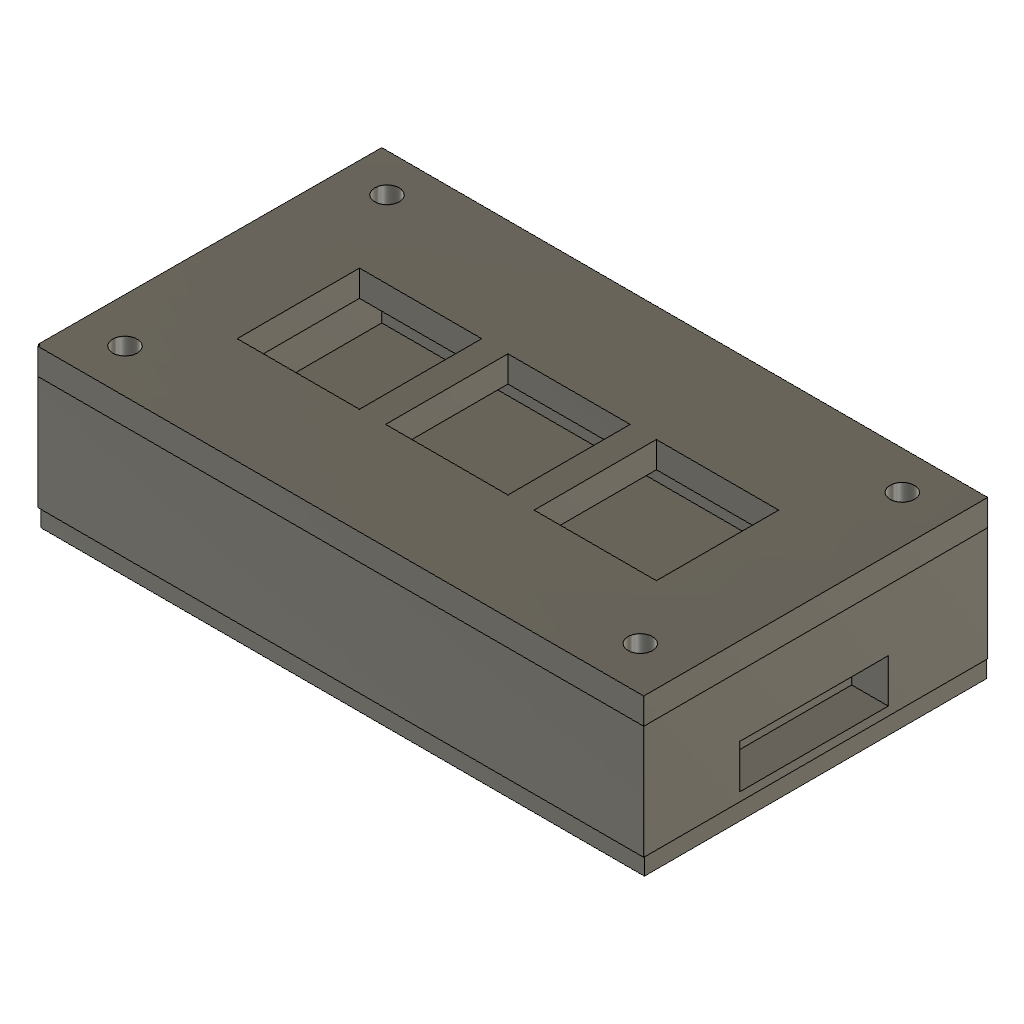
F3D UPDATED (Autodesk Fusion 360 design; units mm, degrees)
part number: 2026-07-22-23-07-19-402
Autodesk Fusion 360 part; units mm, degrees
form "Form1" [no effect]
sketch "sketch 359" plane through (0, 0, 0) normal (0, 0, 1) x (1, 0, 0)
  line L0 (0, 0) -> (49.4, 0)
  line L1 (49.4, 0) -> (49.4, 19.4)
  line L2 (49.4, 19.4) -> (0, 19.4)
  line L3 (0, 19.4) -> (0, 0)
  line L4 (-10, 29.4) -> (59.4, 29.4)
  line L5 (59.4, 29.4) -> (59.4, -10)
  line L6 (59.4, -10) -> (-10, -10)
  line L7 (-10, -10) -> (-10, 29.4)
  circle A0 centre (-5, 25) radius 1.45
  circle A1 centre (54, 25) radius 1.45
  circle A2 centre (54, -5) radius 1.45
  circle A3 centre (-5, -5) radius 1.45
  constraint horizontal L0
  constraint vertical L1
  constraint horizontal L2
  constraint vertical L3
  constraint coincident L0.start L3.end
  constraint horizontal L4
  constraint vertical L5
  constraint horizontal L6
  constraint vertical L7
extrude "Extrude1" add sketch "sketch 359" along normal blind 3 makes body 1
extrude "Extrude2" add 1 faces at (16.3333, 23.5528, 3) along direction (0, 0, 1) blind 10 on bodies 1 bodies 1
sketch "Sketch1" plane through (0, 0, 0) normal (0, 0, 1) x (1, 0, 0)
  line L0 (59.352, 29) -> (-10, 29)
  line L1 (-10, 29) -> (-10, -9.736)
  line L2 (-10, -9.736) -> (59.352, -9.736)
  line L3 (59.352, -9.736) -> (59.352, 29)
  constraint horizontal L0
  constraint vertical L1
  constraint horizontal L2
  constraint vertical L3
extrude "Extrude3" add sketch "Sketch1" along normal blind 3 bodies 1
extrude "Extrude4" cut sketch "sketch 359" along normal through all contours A0 | A1 | A2 | A3 bodies 1
sketch "Sketch2" plane through (0, 0, 3) normal (0, 0, 1) x (-1, 0, 0)
  line L0 (0, 0) -> (-49.4, 0)
  line L1 (-49.4, 0) -> (-49.4, -19.4)
  line L2 (-49.4, -19.4) -> (0, -19.4)
  line L3 (0, -19.4) -> (0, 0)
sketch "Sketch3" plane through (0, 0, 0) normal (0, 0, 1) x (1, 0, 0)
sketch "sketch 3672" plane through (0, 0, 0) normal (0, 0, 1) x (1, 0, 0)
  line L0 (14.5, 16) -> (14.5, 3)
  line L1 (3.0489, 16.475) -> (14, 16.5)
  line L2 (3.025, 2.3766) -> (14, 2.5)
  line L3 (2.5489, 15.975) -> (2.525, 2.8766)
  line L4 (35.3489, 16.4816) -> (46.1543, 16.5621)
  arc A0 (14.5, 16) -> (14, 16.5) centre (14, 16) ccw
  line L5 (30.5, 16) -> (30.5, 3)
  arc A1 (18.5, 3) -> (19, 2.5) centre (19, 3) ccw
  line L6 (18.5, 16) -> (18.5, 3)
  line L7 (35.5886, 2.1369) -> (46.2741, 2.1163)
  line L8 (34.8489, 15.9816) -> (35.0886, 2.6369)
  arc A2 (14, 2.5) -> (14.5, 3) centre (14, 3) ccw
  line L9 (46.6543, 16.0621) -> (46.7741, 2.6163)
  arc A3 (2.525, 2.8766) -> (3.025, 2.3766) centre (3.025, 2.8766) ccw
  arc A4 (3.0489, 16.475) -> (2.5489, 15.975) centre (3.0489, 15.975) ccw
  line L10 (19, 16.5) -> (30, 16.5)
  arc A5 (30.5, 16) -> (30, 16.5) centre (30, 16) ccw
  line L11 (19, 2.5) -> (30, 2.5)
  arc A6 (19, 16.5) -> (18.5, 16) centre (19, 16) ccw
  arc A7 (30, 2.5) -> (30.5, 3) centre (30, 3) ccw
  arc A8 (35.3489, 16.4816) -> (34.8489, 15.9816) centre (35.3489, 15.9816) ccw
  arc A9 (35.0886, 2.6369) -> (35.5886, 2.1369) centre (35.5886, 2.6369) ccw
  arc A10 (46.6543, 16.0621) -> (46.1543, 16.5621) centre (46.1543, 16.0621) ccw
  arc A11 (46.2741, 2.1163) -> (46.7741, 2.6163) centre (46.2741, 2.6163) ccw
  line L12 (-10.0721, -9.8522) -> (-9.8977, 29.2855)
  line L13 (59, -10) -> (59, 29)
  line L14 (-9.8977, 29.2855) -> (59, 29)
  line L15 (-10.0721, -9.8522) -> (59, -10)
extrude "Extrude5" add sketch "sketch 3672" against normal blind 3 separate body makes body 2
sketch "Sketch4" plane through (59.4, 0, 0) normal (1, 0, 0) x (0, 1, 0)
  line L0 (-10, 0) -> (29.4, 0)
  line L1 (29.4, 0) -> (29.4, 13)
  line L2 (29.4, 13) -> (-10, 13)
  line L3 (-10, 13) -> (-10, 0)
  line L4 (1, 9) -> (18, 9)
  line L5 (18, 9) -> (18, 4)
  line L6 (18, 4) -> (1, 4)
  line L7 (1, 4) -> (1, 9)
  dimension "d10" = 5
  dimension "d11" = 17
  constraint horizontal L4
  constraint vertical L5
  constraint horizontal L6
  constraint vertical L7
  measures "d10" distance of L4.end L5.end
  measures "d11" distance of L4.start L4.end
extrude "Extrude6" cut sketch "Sketch4" against normal blind 10 contours L4 L5 L6 L7 bodies 1
sketch "Sketch5" plane through (0, 0, 13) normal (0, 0, 1) x (-1, 0, 0)
  line L0 (0, 0) -> (0, -19.4)
  line L1 (0, -19.4) -> (-49.4, -19.4)
  line L2 (-49.4, -19.4) -> (-49.4, 0)
  line L3 (-49.4, 0) -> (0, 0)
  circle A0 centre (-54, 5) radius 1.45
  circle A1 centre (5, 5) radius 1.45
  circle A2 centre (5, -25) radius 1.45
  circle A3 centre (-54, -25) radius 1.45
  line L4 (10, 10) -> (-59.4, 10)
  line L5 (-59.4, 10) -> (-59.4, -29.4)
  line L6 (-59.4, -29.4) -> (10, -29.4)
  line L7 (10, -29.4) -> (10, 10)
sketch "Sketch6" plane through (0, 0, -3) normal (0, 0, -1) x (1, 0, 0)
  arc A0 (18.5, -16) -> (19, -16.5) centre (19, -16) ccw
  line L0 (18.5, -16) -> (18.5, -3)
  arc A1 (19, -2.5) -> (18.5, -3) centre (19, -3) ccw
  line L1 (19, -2.5) -> (30, -2.5)
  arc A2 (30.5, -3) -> (30, -2.5) centre (30, -3) ccw
  line L2 (30.5, -3) -> (30.5, -16)
  arc A3 (30, -16.5) -> (30.5, -16) centre (30, -16) ccw
  line L3 (30, -16.5) -> (19, -16.5)
  arc A4 (34.8489, -15.9816) -> (35.3489, -16.4816) centre (35.3489, -15.9816) ccw
  line L4 (34.8489, -15.9816) -> (35.0886, -2.6369)
  arc A5 (35.5886, -2.1369) -> (35.0886, -2.6369) centre (35.5886, -2.6369) ccw
  line L5 (35.5886, -2.1369) -> (46.2741, -2.1163)
  arc A6 (46.7741, -2.6163) -> (46.2741, -2.1163) centre (46.2741, -2.6163) ccw
  line L6 (46.7741, -2.6163) -> (46.6543, -16.0621)
  arc A7 (46.1543, -16.5621) -> (46.6543, -16.0621) centre (46.1543, -16.0621) ccw
  line L7 (46.1543, -16.5621) -> (35.3489, -16.4816)
  arc A8 (14, -16.5) -> (14.5, -16) centre (14, -16) ccw
  line L8 (14, -16.5) -> (3.0489, -16.475)
  arc A9 (2.5489, -15.975) -> (3.0489, -16.475) centre (3.0489, -15.975) ccw
  line L9 (2.5489, -15.975) -> (2.525, -2.8766)
  arc A10 (3.025, -2.3766) -> (2.525, -2.8766) centre (3.025, -2.8766) ccw
  line L10 (3.025, -2.3766) -> (14, -2.5)
  arc A11 (14.5, -3) -> (14, -2.5) centre (14, -3) ccw
  line L11 (14.5, -3) -> (14.5, -16)
  line L12 (-10.0721, 9.8522) -> (-9.8977, -29.2855)
  line L13 (-9.8977, -29.2855) -> (59, -29)
  line L14 (59, -29) -> (59, 10)
  line L15 (59, 10) -> (-10.0721, 9.8522)
move_face "MoveFace1" by (-60, 0, 0) 1 faces at (16.3333, 23.5528, 13) on bodies 1
move_face "MoveFace2" to x (0.939693, -0.34202, 0) y (0.34202, 0.939693, 0) z (0, 0, 1) at (-4.6871, -1.2103, -13) 2 faces at (32.9333, 6.4667, 3) (16.3333, 23.5528, 13) on bodies 1
move_body "Move1" bodies 1 to x (1, 0, 0) y (0, 1, 0) z (0, 0, 1) at (-70.6858, -0.1603, 0)
extrude "Extrude7" cut 1 faces at (-36.7879, 5.0494, 0) along direction (0, 0, 1) blind 3 on bodies 1 bodies 1
extrude "Extrude8" add 1 faces at (-54.3524, 23.3925, 13) along direction (0, 0, 1) blind 3 on bodies 1 bodies 1
move_face "MoveFace3" by (-60.7884, -19.4774, 0) 1 faces at (26.3674, 24.9285, 0) on bodies 2
move_face "MoveFace4" by (80, 0, 0) 1 faces at (-54.3524, 23.3925, 16) on bodies 1
move_face "MoveFace5" by (0, 0, 25) 1 faces at (12.9519, -9.9014, -1) on bodies 2
sketch "Sketch7" plane through (0, -10.1603, 0) normal (0, -1, 0) x (1, 0, 0)
  line L0 (-80.6858, 3) -> (-11.2858, 3)
  line L1 (-11.2858, 3) -> (-11.2858, 16)
  line L2 (-11.2858, 16) -> (-80.6858, 16)
  line L3 (-80.6858, 16) -> (-80.6858, 3)
move_face "MoveFace6" by (70, 0, 0) 1 faces at (-54.3524, 23.3925, 16) on bodies 1
move_body "Move2" bodies 2 to x (1, 0, 0) y (0, 1, 0) z (0, 0, 1) at (-70.8, 0, 0)
move_face "MoveFace7" by (0, 0, 20) 1 faces at (-57.8481, -9.9014, -2) on bodies 2
move_body "Move3" bodies 2 to x (1, 0, 0) y (0, 1, 0) z (0, 0, 1) at (0.5, -0.0011, 19)
sketch "Sketch8" plane through (0, 0, 3) normal (0, 0, -1) x (1, 0, 0)
  line L0 (-21.2858, -19.2397) -> (-70.6858, -19.2397)
  line L1 (-70.6858, -19.2397) -> (-70.6858, 0.1603)
  line L2 (-70.6858, 0.1603) -> (-21.2858, 0.1603)
  line L3 (-21.2858, 0.1603) -> (-21.2858, -19.2397)
  circle A0 centre (-16.6858, -24.8397) radius 1.45
  circle A1 centre (-16.6858, 5.1603) radius 1.45
  circle A2 centre (-75.6858, -24.8397) radius 1.45
  circle A3 centre (-75.6858, 5.1603) radius 1.45
  line L4 (-80.6858, 10.1603) -> (-80.6858, -29.2397)
  line L5 (-80.6858, -29.2397) -> (-11.2858, -29.2397)
  line L6 (-11.2858, -29.2397) -> (-11.2858, 10.1603)
  line L7 (-11.2858, 10.1603) -> (-80.6858, 10.1603)
sketch "Sketch9" plane through (0, 0, 3) normal (0, 0, -1) x (1, 0, 0)
sketch "Sketch10" plane through (0, 0, 3) normal (0, 0, -1) x (1, 0, 0)
extrude "Extrude9" add sketch "Sketch8" against normal blind 0.01 contours L0 L1 L2 L3 bodies 1
move_body "Move4" bodies 2 to x (1, 0, 0) y (0, 1, 0) z (0, 0, 1) at (-0.3136, -0.3071, -3)
move_body "Move5" bodies 2 to x (1, 0, 0) y (0, 1, 0) z (0, 0, 1) at (-0.1744, 0.2623, 0)
hole "Hole1" at (-16.6858, 24.8397, 3) direction (0, 0, 1) diameter 2.8 depth 13 tip angle 118 bodies 2
hole "Hole2" at (-16.6858, -5.1603, 3) direction (0, 0, 1) diameter 2.8 depth 13 tip angle 118 bodies 2
hole "Hole3" at (-75.6858, -5.1603, 3) direction (0, 0, 1) diameter 2.8 depth 13 tip angle 118 bodies 2
hole "Hole4" at (-75.6858, 24.8397, 3) direction (0, 0, 1) diameter 2.8 depth 13 tip angle 118 bodies 2
sketch "Sketch11" plane through (0, 0, 16) normal (0, 0, 1) x (-1, 0, 0)
  circle A0 centre (75.6858, -24.8397) radius 1.4
  circle A1 centre (75.6858, 5.1603) radius 1.4
  circle A2 centre (16.6858, 5.1603) radius 1.4
  circle A3 centre (16.6858, -24.8397) radius 1.4
  arc A4 (51.788, -16.4542) -> (52.288, -15.9542) centre (51.788, -15.9542) ccw
  line L0 (51.788, -16.4542) -> (40.788, -16.4542)
  arc A5 (40.288, -15.9542) -> (40.788, -16.4542) centre (40.788, -15.9542) ccw
  line L1 (40.288, -15.9542) -> (40.288, -2.9542)
  arc A6 (40.788, -2.4542) -> (40.288, -2.9542) centre (40.788, -2.9542) ccw
  line L2 (40.788, -2.4542) -> (51.788, -2.4542)
  arc A7 (52.288, -2.9542) -> (51.788, -2.4542) centre (51.788, -2.9542) ccw
  line L3 (52.288, -2.9542) -> (52.288, -15.9542)
  arc A8 (35.4391, -16.4358) -> (35.9391, -15.9358) centre (35.4391, -15.9358) ccw
  line L4 (35.4391, -16.4358) -> (24.6337, -16.5163)
  arc A9 (24.1337, -16.0163) -> (24.6337, -16.5163) centre (24.6337, -16.0163) ccw
  line L5 (24.1337, -16.0163) -> (24.0139, -2.5705)
  arc A10 (24.5139, -2.0705) -> (24.0139, -2.5705) centre (24.5139, -2.5705) ccw
  line L6 (24.5139, -2.0705) -> (35.1994, -2.0911)
  arc A11 (35.6994, -2.5911) -> (35.1994, -2.0911) centre (35.1994, -2.5911) ccw
  line L7 (35.6994, -2.5911) -> (35.9391, -15.9358)
  arc A12 (56.288, -15.9542) -> (56.788, -16.4542) centre (56.788, -15.9542) ccw
  line L8 (56.288, -15.9542) -> (56.288, -2.9542)
  arc A13 (56.788, -2.4542) -> (56.288, -2.9542) centre (56.788, -2.9542) ccw
  line L9 (56.788, -2.4542) -> (67.763, -2.3308)
  arc A14 (68.263, -2.8308) -> (67.763, -2.3308) centre (67.763, -2.8308) ccw
  line L10 (68.263, -2.8308) -> (68.2391, -15.9292)
  arc A15 (67.7391, -16.4292) -> (68.2391, -15.9292) centre (67.7391, -15.9292) ccw
  line L11 (67.7391, -16.4292) -> (56.788, -16.4542)
  line L12 (80.6858, -29.2397) -> (80.8602, 9.898)
  line L13 (80.8602, 9.898) -> (11.788, 10.0458)
  line L14 (11.788, 10.0458) -> (11.788, -28.9542)
  line L15 (11.788, -28.9542) -> (80.6858, -29.2397)
  dimension "d36" = 12
  dimension "d45" = 14
  dimension "d49" = 14.3447
  dimension "d52" = 11.6855
  dimension "d53" = 14.0984
  dimension "d54" = 11.975
  dimension "d56" = 14.4463
  measures "d36" distance of L1 L3
  measures "d45" distance of L0 L2
  measures "d49" vertical distance of A8.start L6.end
  measures "d52" horizontal distance of L5.end A11.start
  measures "d53" vertical distance of L9.end A15.start
  measures "d54" horizontal distance of L8.end A14.start
  measures "d56" distance of L4.end A10.start
sketch "Sketch12" plane through (0, 0, 16) normal (0, 0, 1) x (-1, 0, 0)
  line L0 (70, -16) -> (56, -16)
  line L1 (56, -16) -> (56, -2)
  line L2 (56, -2) -> (70, -2)
  line L3 (70, -2) -> (70, -16)
  line L4 (22, -16) -> (36, -16)
  line L5 (36, -16) -> (36, -2)
  line L6 (36, -2) -> (22, -2)
  line L7 (22, -2) -> (22, -16)
  line L8 (53, -16) -> (39, -16)
  line L9 (39, -16) -> (39, -2)
  line L10 (39, -2) -> (53, -2)
  line L11 (53, -2) -> (53, -16)
  dimension "d57" = 14
  dimension "d58" = 14
  dimension "d59" = 14
  dimension "d60" = 14
  dimension "d61" = 14
  constraint horizontal L0
  constraint vertical L1
  constraint horizontal L2
  constraint vertical L3
  constraint horizontal L4
  constraint vertical L5
  constraint horizontal L6
  constraint vertical L7
  constraint horizontal L8
  constraint vertical L9
  constraint horizontal L10
  constraint vertical L11
  measures "d57" distance of L0.start L0.end
  measures "d58" distance of L4.start L4.end
  measures "d59" distance of L4.start L6.end
  measures "d60" distance of L8.start L8.end
  measures "d61" distance of L8.start L10.end
sketch "Sketch13" plane through (0, 0, 16) normal (0, 0, 1) x (-1, 0, 0)
  line L0 (73, -22) -> (15.4788, -22)
  line L1 (15.4788, -22) -> (15.4788, 2.4214)
  line L2 (15.4788, 2.4214) -> (73, 2.4214)
  line L3 (73, 2.4214) -> (73, -22)
  constraint horizontal L0
  constraint vertical L1
  constraint horizontal L2
  constraint vertical L3
extrude "Extrude10" add sketch "Sketch13" against normal blind 13 bodies 1 2
shell "Shell1" thickness 1.5 removed faces 1 at (-36.7879, 14.63, 3) on bodies 1
extrude "Extrude11" cut sketch "Sketch12" against normal blind 6 bodies 1
extrude "Extrude12" add 1 faces at (-48.4572, 22.5773, 16) along direction (0, 0, 1) blind 3 on bodies 1 bodies 1
sketch "Sketch14" plane through (0, 0, 0) normal (0, 0, 1) x (1, 0, 0)
  line L0 (-80.5, -10, 3) -> (-11.3436, -10, 3)
  line L1 (-11.3436, -10, 3) -> (-11.3436, 29.1649, 3)
  line L2 (-11.3436, 29.1649, 3) -> (-80.5, 29.1649, 3)
  line L3 (-80.5, 29.1649, 3) -> (-80.5, -10, 3)
  line L4 (-80.6858, -10.1603, 3) -> (-11.2858, -10.1603, 3)
  line L5 (-11.2858, -10.1603, 3) -> (-11.2858, 29.2397, 3)
  line L6 (-11.2858, 29.2397, 3) -> (-80.6858, 29.2397, 3)
  line L7 (-80.6858, 29.2397, 3) -> (-80.6858, -10.1603, 3)
  line L8 (-80.6858, -10.1603, 3) -> (-11.2858, -10.1603, 3)
  line L9 (-11.2858, -10.1603, 3) -> (-11.2858, 29.2397, 3)
  line L10 (-11.2858, 29.2397, 3) -> (-80.6858, 29.2397, 3)
  line L11 (-80.6858, 29.2397, 3) -> (-80.6858, -10.1603, 3)
  line L12 (-80.6858, -10.1603, 3) -> (-11.2858, -10.1603, 3)
  line L13 (-11.2858, -10.1603, 3) -> (-11.2858, 29.2397, 3)
  line L14 (-11.2858, 29.2397, 3) -> (-80.6858, 29.2397, 3)
  line L15 (-80.6858, 29.2397, 3) -> (-80.6858, -10.1603, 3)
  line L16 (-80.5, -10) -> (-11.3694, -10)
  line L17 (-11.3694, -10) -> (-11.3694, 29.2038)
  line L18 (-11.3694, 29.2038) -> (-80.5, 29.2038)
  line L19 (-80.5, 29.2038) -> (-80.5, -10)
  point P0 (-80.6858, -10.1603)
  point P1 (-11.2858, 29.2397)
  point P2 (-80.6858, -10.1603)
  point P3 (-11.2858, 29.2397)
  point P4 (-80.6858, -10.1603)
  point P5 (-11.2858, 29.2397)
  constraint coincident P5 P3
  constraint coincident P4 P2
  constraint horizontal L16
  constraint vertical L17
  constraint horizontal L18
  constraint vertical L19
extrude "Extrude13" add sketch "Sketch14" along normal blind 0.1 separate body makes body 3
move_body "Move6" bodies 3 to x (1, 0, 0) y (0, 1, 0) z (0, 0, 1) at (0, 0, 3)
delete_face "DeleteFace1" 1 faces at (-73.7261, 27.0448, 6.8333) on bodies 1
delete_face "DeleteFace2" 1 faces at (-18.9489, 26.732, 6.8333) on bodies 1
delete_face "DeleteFace3" 1 faces at (-75.7593, -2.2112, 10.6667) on bodies 1
delete_face "DeleteFace4" 1 faces at (-13.7504, -4.8666, 10.6667) on bodies 1
sketch "Sketch15" plane through (0, 0, 0) normal (0, 0, 1) x (1, 0, 0)
extrude "Extrude14" cut 1 faces at (-48.4572, 22.5773, 19) along direction (0, 0, -1) blind 1.5 on bodies 1 bodies 1
ref_plane "WorkPlane1" through (-46.073, 9.5397, 14.5) normal (0, 0, 1) x (1, 0, 0)
split "Split1" by plane through (-46.073, 9.5397, 14.5) normal (0, 0, 1) bodies 1 makes body 4 at (-48.4572, 22.5773, 17.5)
move_face "MoveFace8" by (0, 0, -1.5) 2 faces at (-57.5524, -10.1603, 6.8333) (-11.2858, 25.4397, 8.8333) on bodies 1
move_body "Move7" bodies 4 to x (1, 0, 0) y (0, 1, 0) z (0, 0, 1) at (-73, 0, 0)
move_face "OffsetFaces1" offset 1.5 1 faces at (-79.7439, 3.0605, 14.5) on bodies 1
move_body "Move8" bodies 4 to x (1, 0, 0) y (0, 1, 0) z (0, 0, 1) at (73, 0, 1.5)
extrude "Extrude15" add 1 faces at (-57.4565, 16.1359, 3) along direction (0, 0, -1) blind 2 on bodies 3 bodies 1 4 3
